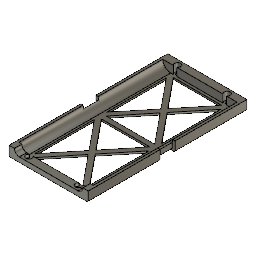
Poweradd Pilot (Autodesk Fusion 360 design; units mm, degrees)
Autodesk Fusion 360 part; units mm, degrees
sketch "スケッチ1" plane through (0, 0, 0) normal (0, 1, 0) x (1, 0, 0)
  line L0 (37.5, -8) -> (-37.5, -8)
  line L1 (-37.5, -8) -> (-37.5, 8)
  line L2 (-37.5, 8) -> (37.5, 8)
  line L3 (37.5, 8) -> (37.5, -8)
  line L4 (37.5, -8) -> (-37.5, 8) construction
  line L5 (-37.5, -8) -> (37.5, 8) construction
  circle A0 centre (-29.5, 0) radius 8
  circle A1 centre (29.5, 0) radius 8
  dimension "d1" = 75
  dimension "d2" = 16
  dimension "d13" = 16
  dimension "d14" = 16
  constraint perpendicular L0 L1
  constraint parallel L0 L2
  constraint parallel L1 L3
  constraint horizontal L0
  constraint coincident L4 origin
  constraint coincident L5 origin
  constraint tangent L0 A0
  constraint tangent L0 A1
  constraint tangent L1 A0
  constraint tangent L3 A1
  measures "d1" distance of L1.end L2.end
  measures "d2" distance of L0.end L1.end
  measures "d13" diameter of A0
  measures "d14" diameter of A1
extrude "押し出し1" add sketch "スケッチ1" along normal mid plane 146 contours L0 L2 A0 A1 | A1 | A0 makes body 1
copy_body "ボディ -> コンポーネント1" bodies 1 removing the originals makes body 2 in component "Component"
sketch "スケッチ2" plane through (0, 0, 0) normal (0, 0, 1) x (1, 0, 0)
  line L0 (25, 75) -> (-25, 75) construction
  line L1 (-25, 75) -> (-25, -75) construction
  line L2 (-25, -75) -> (25, -75) construction
  line L3 (25, -75) -> (25, 75) construction
  line L4 (25, 75) -> (-25, -75) construction
  line L5 (-25, 75) -> (25, -75) construction
  line L6 (36.5, 72) -> (-36.5, 72) construction
  line L7 (-36.5, 72) -> (-36.5, -72) construction
  line L8 (-36.5, -72) -> (36.5, -72) construction
  line L9 (36.5, -72) -> (36.5, 72) construction
  line L10 (36.5, 72) -> (-36.5, -72) construction
  line L11 (-36.5, 72) -> (36.5, -72) construction
  line L12 (40, 80) -> (-40, 80)
  line L13 (-40, 80) -> (-40, -80)
  line L14 (-40, -80) -> (40, -80)
  line L15 (40, -80) -> (40, 80)
  line L16 (40, 80) -> (-40, -80) construction
  line L17 (-40, 80) -> (40, -80) construction
  dimension "d5" = 150
  dimension "d6" = 50
  dimension "d7" = 73
  dimension "d8" = 144
  dimension "d9" = 80
  dimension "d10" = 160
  constraint perpendicular L0 L1
  constraint parallel L0 L2
  constraint parallel L1 L3
  constraint horizontal L0
  constraint coincident L4 origin
  constraint coincident L5 origin
  constraint perpendicular L6 L7
  constraint parallel L6 L8
  constraint parallel L7 L9
  constraint horizontal L6
  constraint coincident L10 origin
  constraint coincident L11 origin
  constraint perpendicular L12 L13
  constraint parallel L12 L14
  constraint parallel L13 L15
  constraint horizontal L12
  constraint coincident L16 origin
  constraint coincident L17 origin
  measures "d5" distance of L0.end L1.end
  measures "d6" distance of L1.end L2.end
  measures "d7" distance of L7.end L8.end
  measures "d8" distance of L6.end L7.end
  measures "d9" distance of L13.end L14.end
  measures "d10" distance of L12.end L13.end
extrude "押し出し2" add sketch "スケッチ2" against normal blind 10 separate body makes body 3
combine "結合1" operation cut target body 3 tool bodies 2
sketch "スケッチ3" plane through (0, 0, -10) normal (0, 0, -1) x (-1, 0, 0)
  line L0 (-40, 80) -> (-40, -80)
  line L1 (40, 80) -> (-40, 80)
  line L2 (40, -80) -> (40, 80)
  line L3 (-40, -80) -> (40, -80)
  line L4 (25, -75) -> (-25, -75) construction
  line L5 (-25, -75) -> (-25, 75) construction
  line L6 (-25, 75) -> (25, 75) construction
  line L7 (25, 75) -> (25, -75) construction
  line L8 (25, -75) -> (-25, 75) construction
  line L9 (-25, -75) -> (25, 75) construction
  circle A0 centre (25, 75) radius 1.6
  circle A1 centre (-25, 75) radius 1.6
  circle A2 centre (25, -75) radius 1.6
  circle A3 centre (-25, -75) radius 1.6
  dimension "d15" = 150
  dimension "d16" = 50
  dimension "d17" = 3.2
  dimension "d20" = -50
  dimension "d21" = -150
  constraint perpendicular L4 L5
  constraint parallel L4 L6
  constraint parallel L5 L7
  constraint horizontal L4
  constraint coincident L8 origin
  constraint coincident L9 origin
  constraint coincident L6.end L7.start
  measures "d15" distance of L4.end L5.end
  measures "d16" distance of L5.end L6.end
  measures "d17" diameter of A0
extrude "押し出し3" cut sketch "スケッチ3" against normal through all contours A0 | A1 | A2 | A3 bodies 3
sketch "スケッチ6" plane through (0, -73, 0) normal (0, 1, 0) x (-1, 0, 0)
  line L0 (37.5, 0) -> (-37.5, 0)
  arc A0 (-37.5, 0) -> (-29.5, -8) centre (-29.5, 0) ccw
  line L1 (-29.5, -8) -> (29.5, -8)
  arc A1 (29.5, -8) -> (37.5, 0) centre (29.5, 0) ccw
  arc A2 (-34.5, 0) -> (-29.5, -5) centre (-29.5, 0) ccw
  line L2 (-29.5, -5) -> (29.5, -5)
  arc A3 (29.5, -5) -> (34.5, 0) centre (29.5, 0) ccw
  line L3 (-34.5, 0) -> (34.5, 0)
  dimension "d37" = 3
extrude "押し出し7" cut sketch "スケッチ6" against normal through all contours L0 A2 L2 A3 L3 bodies 3
sketch "スケッチ7" plane through (0, 0, 0) normal (0, 0, 1) x (-1, 0, 0)
  line L0 (34.5, 80) -> (34.5, 73)
  line L1 (34.5, 73) -> (37.5, 73)
  line L2 (37.5, 73) -> (37.5, -73)
  line L3 (37.5, -73) -> (-37.5, -73)
  line L4 (-37.5, -73) -> (-37.5, 73)
  line L5 (-37.5, 73) -> (-34.5, 73)
  line L6 (-34.5, 73) -> (-34.5, 80)
  line L7 (-34.5, 80) -> (-40, 80)
  line L8 (-40, 80) -> (-40, -80)
  line L9 (-40, -80) -> (40, -80)
  line L10 (40, -80) -> (40, 80)
  line L11 (40, 80) -> (34.5, 80)
  circle A0 centre (-25, -75) radius 1.6
  circle A1 centre (25, -75) radius 1.6
  circle A2 centre (25, -75) radius 3
  circle A3 centre (-25, -75) radius 3
  dimension "d42" = 6
  dimension "d43" = 6
  constraint concentric A1 A2
  constraint concentric A0 A3
  measures "d42" diameter of A2
  measures "d43" diameter of A3
extrude "押し出し8" cut sketch "スケッチ7" against normal blind 3 contours L3 A2 | L3 A3 picked at (24.9601, -73.1348) picked at (-25.0399, -73.1348) bodies 3
sketch "スケッチ8" plane through (0, 0, -5) normal (0, 0, 1) x (-1, 0, 0)
  circle A0 centre (-25, 75) radius 1.6
  circle A1 centre (25, 75) radius 1.6
  line L0 (29.5, 80) -> (-29.5, 80)
  line L1 (-29.5, 80) -> (-29.5, 73)
  line L2 (-29.5, 73) -> (29.5, 73)
  line L3 (29.5, 73) -> (29.5, 80)
  circle A2 centre (-25, 75) radius 3
  circle A3 centre (25, 75) radius 3
  dimension "d46" = 6
  dimension "d47" = 6
  constraint concentric A0 A2
  constraint concentric A1 A3
  measures "d46" diameter of A2
  measures "d47" diameter of A3
extrude "押し出し9" cut sketch "スケッチ8" against normal blind 2 contours L2 A3 | L2 A2 picked at (24.9601, 73.1348) picked at (-25.0399, 73.1348) bodies 3
sketch "スケッチ9" plane through (0, 0, 0) normal (0, 1, 0) x (1, 0, 0)
  line L0 (40, 0) -> (37, 0)
  line L1 (37, 0) -> (37, 10)
  line L2 (37, 10) -> (40, 10)
  line L3 (40, 10) -> (40, 0)
  line L4 (-40, 10) -> (40, 10)
  line L5 (40, 10) -> (34, 10)
  line L6 (34, 10) -> (34, 10.0001)
  line L7 (34, 10.0001) -> (40, 10.0001)
  line L8 (40, 10.0001) -> (40, 10)
  line L9 (-37, 0) -> (-40, 0)
  line L10 (-40, 0) -> (-40, 10)
  line L11 (-40, 10) -> (-37, 10)
  line L12 (-37, 10) -> (-37, 0)
  line L13 (-40, 10) -> (-34, 10)
  line L14 (-34, 10) -> (-34, 8)
  line L15 (-34, 8) -> (-40, 8)
  line L16 (-40, 8) -> (-40, 10)
  line L17 (0, 0) -> (0, 10) construction
  line L18 (34, 8) -> (40, 8)
  line L19 (34, 10) -> (34, 8)
  point P0 (40, 0)
  dimension "d50" = 6
  dimension "d51" = 2
  constraint horizontal L0
  constraint vertical L1
  constraint horizontal L2
  constraint vertical L3
  constraint coincident L1.end L4
  constraint coincident P0 L0.start
  constraint horizontal L5
  constraint vertical L6
  constraint horizontal L7
  constraint vertical L8
  constraint coincident L2.end L3.start
  constraint horizontal L9
  constraint vertical L10
  constraint horizontal L11
  constraint vertical L12
  constraint coincident L4.start L10.end
  constraint horizontal L13
  constraint vertical L14
  constraint horizontal L15
  constraint vertical L16
  constraint coincident L17.start origin
  constraint midpoint L4 L17.end
  constraint symmetric L13.end L17 L5.end
  constraint symmetric L14.end L17 L18.start
  constraint symmetric L15.end L17 L18.end
  measures "d50" distance of L4.start L13.end
  measures "d51" distance of L4.start L15.end
extrude "押し出し10" cut sketch "スケッチ9" along normal mid plane 15 bodies 3
sketch "スケッチ10" plane through (0, 0, 0) normal (0, 1, 0) x (1, 0, 0)
  arc A0 (-29.5, 8) -> (-37.5, 0) centre (-29.5, 0) ccw
  arc A1 (-29.5, 5) -> (-34.5, 0) centre (-29.5, 0) ccw
  line L0 (-34.5, 0) -> (-40, 0)
  line L1 (-40, 0) -> (-40, 10)
  line L2 (-40, 10) -> (40, 10)
  line L3 (40, 10) -> (40, 0)
  line L4 (40, 0) -> (34.5, 0)
  arc A2 (34.5, 0) -> (29.5, 5) centre (29.5, 0) ccw
  line L5 (29.5, 5) -> (-29.5, 5)
  arc A3 (-29.5, 8) -> (-37.5, 0) centre (-29.5, 0) ccw
  line L6 (29.5, 8) -> (-29.5, 8)
  line L7 (-29.5, 8) -> (29.5, 8)
  arc A4 (-29.5, 8) -> (-37.5, 0) centre (-29.5, 0) ccw
  line L8 (-29.5, 8) -> (29.5, 8)
  line L9 (0, 0) -> (-40, 0)
  line L10 (29.5, -8) -> (-29.5, -8)
  arc A5 (-37.5, 0) -> (-29.5, -8) centre (-29.5, 0) ccw
  line L11 (-37.5, 0) -> (-36.672, 9.4638)
  line L12 (-37.5, 0) -> (-26.5, 0) construction
  line L13 (-36.672, 9.4638) -> (-34.6982, 9.1414)
  line L14 (-34.6982, 9.1414) -> (-34.4564, 10.6218)
  line L15 (-34.6982, 9.1414) -> (-31.2071, 9.1414) construction
  line L16 (0, -8) -> (0, 10) construction
  arc A6 (29.5, -8) -> (37.5, 0) centre (29.5, 0) ccw
  line L17 (37.5, 0) -> (36.672, 9.4639)
  line L18 (34.6982, 9.1414) -> (34.4564, 10.6218)
  line L19 (36.672, 9.4639) -> (34.6982, 9.1414)
  line L20 (-38.0254, 11.2048) -> (-34.4564, 10.6218)
  line L21 (-38.9998, 0.0683) -> (-38.0254, 11.2048)
  arc A7 (-38.9998, 0.0683) -> (-29.5, -9.5) centre (-29.5, 0) ccw
  line L22 (29.5, -9.5) -> (-29.5, -9.5)
  arc A8 (29.5, -9.5) -> (38.9998, 0.0683) centre (29.5, 0) ccw
  line L23 (38.9998, 0.0683) -> (38.0254, 11.2048)
  line L24 (38.0254, 11.2048) -> (34.4564, 10.6218)
  line L25 (28.5, -9.5) -> (-28.5, -9.5) construction
  line L26 (-28.5, -9.5) -> (-28.5, -6.5)
  line L27 (-28.5, -6.5) -> (28.5, -6.5) construction
  line L28 (28.5, -6.5) -> (28.5, -9.5)
  line L29 (28.5, -9.5) -> (-28.5, -6.5) construction
  line L30 (-28.5, -9.5) -> (28.5, -6.5) construction
  line L31 (30, -11) -> (-30, -11)
  line L32 (-30, -11) -> (-30, -5)
  line L33 (-30, -5) -> (30, -5)
  line L34 (30, -5) -> (30, -11)
  line L35 (30, -11) -> (-30, -5) construction
  line L36 (-30, -11) -> (30, -5) construction
  point P0 (0, -8)
  point P1 (0, -8)
  dimension "d54" = 85
  dimension "d55" = 9.5
  dimension "d56" = 2
  dimension "d59" = 1.5
  dimension "d70" = 57
  dimension "d71" = 3
  dimension "d72" = 60
  dimension "d73" = 6
  constraint coincident L9.start origin
  constraint coincident L0.end L1.start
  constraint symmetric A0.start L9 L10.end
  constraint symmetric A0.end L9 A3.end
  constraint symmetric A0 L9 A5
  constraint symmetric L6.start L9 L10.start
  constraint coincident A0.end A3.end
  constraint horizontal L12
  constraint horizontal L15
  constraint midpoint L10 P1
  constraint midpoint L2 L16.end
  constraint symmetric L10.end L16 L10.start
  constraint symmetric A0.end L16 A6.end
  constraint symmetric A5 L16 A6
  constraint symmetric L11.end L16 L17.end
  constraint symmetric L13.end L16 L18.start
  constraint symmetric L16 L18.end L14.end
  constraint perpendicular L25 L26
  constraint parallel L25 L27
  constraint parallel L26 L28
  constraint horizontal L25
  constraint coincident L29 P1
  constraint coincident L30 P1
  constraint coincident P1 P0
  constraint perpendicular L31 L32
  constraint parallel L31 L33
  constraint parallel L32 L34
  constraint horizontal L31
  constraint coincident L35 P1
  constraint coincident L36 P1
  measures "d54" angle of L11 L12
  measures "d55" distance of A0.end L11.end
  measures "d56" distance of L11.end L13.end
  measures "d70" distance of L26.end L27.end
  measures "d71" distance of L25.end L26.end
  measures "d72" distance of L32.end L33.end
  measures "d73" distance of L31.end L32.end
extrude "押し出し1'" add sketch "スケッチ10" along normal mid plane 14.5 separate body contours A0 L0 L2 A3 A4 L9 L11 L13 L14 L21 A7 | L0 L9 A5 A7 L32 | L10 A5 A7 L22 L26 L32 | A7 L22 A8 L31 L32 L34 | L2 L14 L20 L21 | L2 L18 L23 L24 | L2 L4 L17 L18 L19 A8 L23 | L10 A6 L22 A8 L28 L34 | L4 A6 A8 L34 makes body 4 in component "Component'"
sketch "スケッチ11" plane through (0, 0, -8) normal (0, 0, 1) x (-1, 0, 0)
  line L0 (29.5, -73) -> (29.5, 73)
  line L1 (29.5, 73) -> (-29.5, 73)
  line L2 (-29.5, 73) -> (-29.5, -73)
  line L3 (-29.5, -73) -> (29.5, -73)
  line L4 (-27.5, -70) -> (27.5, -70)
  line L5 (27.5, -70) -> (27.5, 70)
  line L6 (27.5, 70) -> (-27.5, 70)
  line L7 (-27.5, 70) -> (-27.5, -70)
  line L8 (-27.5, -70) -> (27.5, 70) construction
  line L9 (27.5, -70) -> (-27.5, 70) construction
  line L10 (-27.5, 2.5) -> (27.5, 2.5)
  line L11 (27.5, 2.5) -> (27.5, -2.5)
  line L12 (27.5, -2.5) -> (-27.5, -2.5)
  line L13 (-27.5, -2.5) -> (-27.5, 2.5)
  line L14 (-27.5, 2.5) -> (27.5, -2.5) construction
  line L15 (27.5, 2.5) -> (-27.5, -2.5) construction
  line L16 (27.5, -2.5) -> (-27.5, -70)
  line L17 (27.5, -70) -> (-27.5, -2.5)
  line L18 (25.5619, -0.9208) -> (-29.4381, -68.4208)
  line L19 (29.4381, -4.0792) -> (-25.5619, -71.5792)
  line L20 (29.4381, -68.4208) -> (-25.5619, -0.9208)
  line L21 (25.5619, -71.5792) -> (-29.4381, -4.0792)
  line L22 (27.5, 0) -> (-27.5, 0)
  line L23 (29.4381, 68.4208) -> (-25.5619, 0.9208)
  line L24 (25.5619, 71.5792) -> (-29.4381, 4.0792)
  line L25 (29.4381, 4.0792) -> (-25.5619, 71.5792)
  line L26 (25.5619, 0.9208) -> (-29.4381, 68.4208)
  dimension "d62" = 140
  dimension "d63" = 55
  dimension "d64" = 5
  dimension "d65" = 2.5
  dimension "d66" = 2.5
  dimension "d67" = 2.5
  dimension "d68" = 2.5
  constraint perpendicular L4 L5
  constraint parallel L4 L6
  constraint parallel L5 L7
  constraint horizontal L4
  constraint coincident L8 origin
  constraint coincident L9 origin
  constraint perpendicular L10 L11
  constraint parallel L10 L12
  constraint parallel L11 L13
  constraint horizontal L10
  constraint coincident L7 L10.start
  constraint coincident L14 origin
  constraint coincident L15 origin
  constraint midpoint L5 L22.start
  constraint midpoint L7 L22.end
  constraint symmetric L18.start L22 L26.start
  constraint symmetric L18.end L22 L26.end
  constraint symmetric L19.start L22 L25.start
  constraint symmetric L19.end L22 L25.end
  constraint symmetric L20.start L22 L23.start
  constraint symmetric L20.end L22 L23.end
  constraint symmetric L21.start L22 L24.start
  constraint symmetric L21.end L22 L24.end
  measures "d62" distance of L4.end L5.end
  measures "d63" distance of L5.end L6.end
  measures "d64" distance of L10.end L11.end
extrude "押し出し11" cut sketch "スケッチ11" against normal through all contours L4 L19 L21 | L7 L18 L21 | L5 L19 L20 | L12 L18 L20 | L7 L24 L26 | L10 L23 L26 | L5 L23 L25 | L6 L24 L25 bodies 3
fillet "フィレット1" radius 3 4 edges at (30, 0, 9.4868) (30, 0, 11) (-30, 0, 9.4868) (-30, 0, 11) on bodies 4 in component "Component'"
extrude "押し出し12" cut 1 faces at (-24.9601, 73.1348, -3) along direction (0, 0, -1) blind 4 on bodies 3 bodies 3
extrude "押し出し13" cut 1 faces at (25.0399, 73.1348, -3) along direction (0, 0, -1) blind 4 on bodies 3 bodies 3
extrude "押し出し14" add 1 faces at (25.0399, -73.1348, -7) along direction (0, 0, 1) blind 2 on bodies 3 bodies 3
extrude "押し出し15" add 1 faces at (-24.9601, -73.1348, -7) along direction (0, 0, 1) blind 2 on bodies 3 bodies 3
extrude "押し出し16" add 1 faces at (-9.8333, -73, -7) along direction (0, 1, 0) blind 0.5 on bodies 3 bodies 3
extrude "押し出し17" cut sketch "スケッチ8" against normal blind 2 contours L2 A3 | L2 A3 bodies 3
extrude "押し出し18" cut sketch "スケッチ8" against normal blind 2 contours L2 A2 | L2 A2 bodies 3
extrude "押し出し19" add 2 faces at (-24.9601, 73.1348, -7) (25.0399, 73.1348, -7) along direction (0, 0, 1) blind 7 on bodies 3 bodies 3
extrude "押し出し20" add 1 faces at (-9.8333, 73, -2.6667) along direction (0, -1, 0) blind 0.5 on bodies 3 bodies 3
extrude "押し出し21" cut sketch "スケッチ7" against normal blind 7 contours L3 A2 | L3 A2 bodies 3
extrude "押し出し22" cut sketch "スケッチ7" against normal blind 7 contours L3 A3 | L3 A3 bodies 3
extrude "押し出し23" cut 2 faces at (-25.0399, 72.8015, -7) (25.0399, 72.8015, -7) along direction (0, 0, -1) blind 1 on bodies 3 bodies 3
extrude "押し出し24" cut 2 faces at (24.9601, -72.8015, -7) (-24.9601, -72.8015, -7) along direction (0, 0, -1) blind 1 on bodies 3 bodies 3
chamfer "面取り1" distance 1 angle 45 4 edges at (40, -43.75, -10) (40, 43.75, -10) (-40, 43.75, -10) (-40, -43.75, -10) on bodies 3
component "Component" placed x (1, 0, 0) y (0, 1, 0) z (0, 0, 1) at (0, 0, 0)
component "Component'" placed x (1, 0, 0) y (0, 1, 0) z (0, 0, 1) at (0, 0, 0)
equation "d1 = 73 mm + 2 mm"
equation "d2 = 15 mm + 1 mm"
equation "d13 = d2"
equation "d14 = d13"
